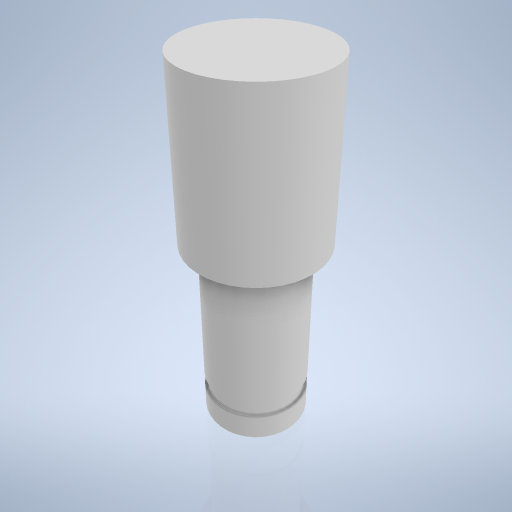
# Autodesk Inventor part: Achse.planetenrad
Saved by Autodesk Inventor 2024.2 (Build 282272000, 272)
## iProperties
Created: 2024-04-30
Part Number: Achse.planetenrad
Material: Generisch
Document SubType Name: Modeling
Designer: Fabri
Density: 1 g/cm^3
Appearance: Vorgabe
Author: Fabri
Autodesk Inventor part; units mm, degrees
ref_plane "YZ Plane" through (0, 0, 0) normal (1, 0, 0) x (0, 1, 0)
ref_plane "XZ Plane" through (0, 0, 0) normal (0, 1, 0) x (-1, 0, 0)
ref_plane "XY Plane" through (0, 0, 0) normal (0, 0, 1) x (1, 0, 0)
sketch "Skizze1" plane through (0, 0, 0) normal (0, 1, 0) x (-1, 0, 0)
  line L0 (0, 0) -> (4, 0)
  line L1 (4, 0) -> (4, -10)
  line L2 (4, -10) -> (3, -10)
  line L3 (3, -10) -> (3, -19)
  line L4 (3, -19) -> (2.85, -19)
  line L5 (2.85, -19) -> (2.85, -19.8)
  line L6 (2.85, -19.8) -> (3, -19.8)
  line L7 (3, -19.8) -> (3, -22)
  line L8 (3, -22) -> (0, -22)
  line L9 (0, -22) -> (0, 0)
  point P0 (1.5, -22)
  dimension "d0" = 10
  dimension "d1" = 22
  dimension "d3" = 9
  dimension "d4" = 0.8
  dimension "d5" = 8
  dimension "d6" = 6
  dimension "d7" = 5.7
  constraints: 20 end point, 8 perpendicular, 2 point on line, 1 horizontal, 1 midpoint
  measures "d0" distance between parallel lines of L0 L2
  measures "d1" distance from line of point (1.5, -22) L0
  measures "d3" distance of L2.end L3.end
  measures "d4" distance between parallel lines of L4 L6
  measures "d5" diameter of L1 L9
  measures "d6" diameter of L3 L9
  measures "d7" diameter of L5 L9
revolve "Umdrehung1" add sketch "Skizze1" angle 360 about axis through (0, 0, -22) along (0, 0, 1)
chamfer "Fasen1" distance 0.5 angle 45 1 edges at (3, 0, -22)
